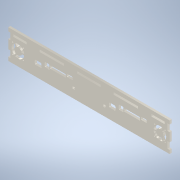
# Autodesk Inventor part: case bottom back
Saved by Autodesk Inventor 2022 (Build 260153000, 153)
## iProperties
Created: 2021-05-28
Part Number: case bottom back
Material: Titanium
Document SubType Name: Modeling
Designer: benka
Density: 4.51 g/cm^3
Appearance: Titanium
Author: benka
Autodesk Inventor part; units mm, degrees
ref_plane "YZ Plane" through (0, 0, 0) normal (1, 0, 0) x (0, 1, 0)
ref_plane "XZ Plane" through (0, 0, 0) normal (0, 1, 0) x (-1, 0, 0)
ref_plane "XY Plane" through (0, 0, 0) normal (0, 0, 1) x (1, 0, 0)
sketch "Sketch1" plane through (0, 0, 0) normal (0, 0, 1) x (1, 0, 0)
  circle A0 centre (-374.8345, 89.3147) radius 3
  line L0 (-376.9823, 107.1342) -> (-376.9823, 104.6342)
  line L1 (-378.9823, 102.6342) -> (-387.9823, 102.6342)
  line L2 (-389.9823, 104.6342) -> (-389.9823, 107.1342)
  line L3 (-392.0636, 104.796) -> (-392.0636, 101.796)
  line L4 (-394.0636, 99.796) -> (-426.0636, 99.796)
  line L5 (-428.0636, 101.796) -> (-428.0636, 104.796)
  line L6 (-429.4023, 105.6169) -> (-429.4023, 99.1169)
  line L7 (-431.4023, 97.1169) -> (-438.2023, 97.1169)
  line L8 (-440.2023, 99.1169) -> (-440.2023, 105.6169)
  line L9 (-447.5294, 98.9881) -> (-447.5294, 92.9881)
  line L10 (-460.5294, 100.9881) -> (-449.5294, 100.9881)
  line L11 (-449.5294, 90.9881) -> (-460.5294, 90.9881)
  line L12 (-462.5294, 92.9881) -> (-462.5294, 98.9881)
  circle A1 centre (-488.8435, 85.8263) radius 1.5
  circle A2 centre (-512.8435, 85.8263) radius 1.5
  circle A3 centre (-512.8435, 109.8263) radius 1.5
  circle A4 centre (-488.8435, 109.8263) radius 1.5
  arc A5 (-486.648, 100.2443) -> (-505.8473, 111.329) centre (-500.8435, 97.8263) ccw
  arc A6 (-505.8473, 111.329) -> (-506.3659, 109.8913) centre (-505.4999, 110.3913) ccw
  line L13 (-503.8384, 105.5136) -> (-506.3659, 109.8913)
  line L14 (-508.5309, 108.6413) -> (-506.0034, 104.2636)
  arc A7 (-508.5309, 108.6413) -> (-510.0353, 108.9111) centre (-509.397, 108.1413) ccw
  arc A8 (-510.0353, 108.9111) -> (-510.0353, 86.7416) centre (-500.8435, 97.8263) ccw
  arc A9 (-506.0034, 104.2636) -> (-506.0034, 91.3891) centre (-500.8435, 97.8263) ccw
  arc A10 (-492.6888, 99.0763) -> (-503.8384, 105.5136) centre (-500.8435, 97.8263) ccw
  line L15 (-487.6338, 99.0763) -> (-492.6888, 99.0763)
  arc A11 (-487.6338, 99.0763) -> (-486.648, 100.2443) centre (-487.6338, 100.0763) ccw
  line L16 (-492.6888, 96.5763) -> (-487.6338, 96.5763)
  arc A12 (-486.648, 95.4084) -> (-487.6338, 96.5763) centre (-487.6338, 95.5763) ccw
  arc A13 (-505.8473, 84.3237) -> (-486.648, 95.4084) centre (-500.8435, 97.8263) ccw
  arc A14 (-503.8384, 90.1391) -> (-492.6888, 96.5763) centre (-500.8435, 97.8263) ccw
  line L17 (-506.3659, 85.7614) -> (-503.8384, 90.1391)
  arc A15 (-506.3659, 85.7614) -> (-505.8473, 84.3237) centre (-505.4999, 85.2614) ccw
  line L18 (-506.0034, 91.3891) -> (-508.5309, 87.0114)
  arc A16 (-510.0353, 86.7416) -> (-508.5309, 87.0114) centre (-509.397, 87.5114) ccw
  line L19 (-438.2023, 107.6169) -> (-431.4023, 107.6169)
  line L20 (-426.0636, 106.796) -> (-394.0636, 106.796)
  line L21 (-387.9823, 109.1342) -> (-378.9823, 109.1342)
  arc A17 (-462.5294, 92.9881) -> (-460.5294, 90.9881) centre (-460.5294, 92.9881) ccw
  arc A18 (-449.5294, 90.9881) -> (-447.5294, 92.9881) centre (-449.5294, 92.9881) ccw
  arc A19 (-447.5294, 98.9881) -> (-449.5294, 100.9881) centre (-449.5294, 98.9881) ccw
  arc A20 (-460.5294, 100.9881) -> (-462.5294, 98.9881) centre (-460.5294, 98.9881) ccw
  arc A21 (-440.2023, 99.1169) -> (-438.2023, 97.1169) centre (-438.2023, 99.1169) ccw
  arc A22 (-431.4023, 97.1169) -> (-429.4023, 99.1169) centre (-431.4023, 99.1169) ccw
  arc A23 (-429.4023, 105.6169) -> (-431.4023, 107.6169) centre (-431.4023, 105.6169) ccw
  arc A24 (-438.2023, 107.6169) -> (-440.2023, 105.6169) centre (-438.2023, 105.6169) ccw
  arc A25 (-428.0636, 101.796) -> (-426.0636, 99.796) centre (-426.0636, 101.796) ccw
  arc A26 (-426.0636, 106.796) -> (-428.0636, 104.796) centre (-426.0636, 104.796) ccw
  arc A27 (-392.0636, 104.796) -> (-394.0636, 106.796) centre (-394.0636, 104.796) ccw
  arc A28 (-394.0636, 99.796) -> (-392.0636, 101.796) centre (-394.0636, 101.796) ccw
  arc A29 (-389.9823, 104.6342) -> (-387.9823, 102.6342) centre (-387.9823, 104.6342) ccw
  arc A30 (-387.9823, 109.1342) -> (-389.9823, 107.1342) centre (-387.9823, 107.1342) ccw
  arc A31 (-376.9823, 107.1342) -> (-378.9823, 109.1342) centre (-378.9823, 107.1342) ccw
  arc A32 (-378.9823, 102.6342) -> (-376.9823, 104.6342) centre (-378.9823, 104.6342) ccw
  line L22 (-522.8987, 75.8147) -> (-522.8987, 67.8147)
  line L23 (-522.8987, 75.8147) -> (-517.8987, 75.8147)
  line L24 (-517.8987, 90.8139) -> (-517.8987, 75.8147)
  line L25 (-522.8987, 90.8139) -> (-517.8987, 90.8139)
  line L26 (-522.8987, 110.8139) -> (-522.8987, 90.8139)
  line L27 (-522.8987, 110.8139) -> (-517.8987, 110.8139)
  line L28 (-522.8987, 125.8154) -> (-517.8987, 125.8154)
  line L29 (-522.8987, 125.8154) -> (-522.8987, 133.8154)
  line L30 (-161.8987, 125.8154) -> (-161.8987, 110.8139)
  line L31 (-161.8987, 110.8139) -> (-156.8987, 110.8139)
  line L32 (-156.8987, 110.8139) -> (-156.8987, 90.8139)
  line L33 (-161.8987, 90.8139) -> (-156.8987, 90.8139)
  line L34 (-161.8987, 90.8139) -> (-161.8987, 75.8147)
  line L35 (-161.8987, 75.8147) -> (-156.8987, 75.8147)
  line L36 (-156.8987, 75.8147) -> (-156.8987, 67.8147)
  line L37 (-161.8987, 125.8154) -> (-156.8987, 125.8154)
  line L38 (-156.8987, 125.8154) -> (-156.8987, 133.8154)
  line L39 (-156.8987, 133.8154) -> (-522.8987, 133.8154)
  line L40 (-522.8987, 67.8147) -> (-156.8987, 67.8147)
  line L41 (-511.3987, 125.8154) -> (-481.3987, 125.8154)
  line L42 (-481.3987, 120.8154) -> (-481.3987, 125.8154)
  line L43 (-511.3987, 120.8154) -> (-481.3987, 120.8154)
  line L44 (-511.3987, 120.8154) -> (-511.3987, 125.8154)
  line L45 (-451.3987, 125.8154) -> (-396.3987, 125.8154)
  line L46 (-451.3987, 120.8154) -> (-451.3987, 125.8154)
  line L47 (-451.3987, 120.8154) -> (-396.3987, 120.8154)
  line L48 (-396.3987, 120.8154) -> (-396.3987, 125.8154)
  line L49 (-366.3987, 120.8154) -> (-366.3987, 125.8154)
  line L50 (-366.3987, 125.8154) -> (-313.3987, 125.8154)
  line L51 (-366.3987, 120.8154) -> (-313.3987, 120.8154)
  line L52 (-313.3987, 120.8154) -> (-313.3987, 125.8154)
  line L53 (-283.3987, 120.8154) -> (-283.3987, 125.8154)
  line L54 (-283.3987, 125.8154) -> (-228.3987, 125.8154)
  line L55 (-283.3987, 120.8154) -> (-228.3987, 120.8154)
  line L56 (-228.3987, 120.8154) -> (-228.3987, 125.8154)
  line L57 (-198.3987, 120.8154) -> (-198.3987, 125.8154)
  line L58 (-198.3987, 125.8154) -> (-168.3987, 125.8154)
  line L59 (-168.3987, 120.8154) -> (-168.3987, 125.8154)
  line L60 (-198.3987, 120.8154) -> (-168.3987, 120.8154)
  circle A33 centre (-304.8345, 89.3147) radius 3
  line L61 (-187.1085, 96.5763) -> (-192.1635, 96.5763)
  line L62 (-192.1635, 99.0763) -> (-187.1085, 99.0763)
  arc A34 (-192.1635, 96.5763) -> (-193.1493, 95.4084) centre (-192.1635, 95.5763) ccw
  arc A35 (-193.1493, 100.2443) -> (-192.1635, 99.0763) centre (-192.1635, 100.0763) ccw
  circle A36 centre (-190.9538, 85.8263) radius 1.5
  circle A37 centre (-190.9538, 109.8263) radius 1.5
  arc A38 (-173.95, 111.329) -> (-193.1493, 100.2443) centre (-178.9538, 97.8263) ccw
  arc A39 (-193.1493, 95.4084) -> (-173.95, 84.3237) centre (-178.9538, 97.8263) ccw
  arc A40 (-175.9589, 105.5136) -> (-187.1085, 99.0763) centre (-178.9538, 97.8263) ccw
  arc A41 (-187.1085, 96.5763) -> (-175.9589, 90.1391) centre (-178.9538, 97.8263) ccw
  line L63 (-173.4314, 85.7614) -> (-175.9589, 90.1391)
  arc A42 (-173.95, 84.3237) -> (-173.4314, 85.7614) centre (-174.2975, 85.2614) ccw
  line L64 (-173.7939, 91.3891) -> (-171.2664, 87.0114)
  arc A43 (-171.2664, 87.0114) -> (-169.762, 86.7416) centre (-170.4003, 87.5114) ccw
  circle A44 centre (-166.9538, 85.8263) radius 1.5
  circle A45 centre (-166.9538, 109.8263) radius 1.5
  arc A46 (-173.4314, 109.8913) -> (-173.95, 111.329) centre (-174.2975, 110.3913) ccw
  line L65 (-175.9589, 105.5136) -> (-173.4314, 109.8913)
  line L66 (-171.2664, 108.6413) -> (-173.7939, 104.2636)
  arc A47 (-169.762, 108.9111) -> (-171.2664, 108.6413) centre (-170.4003, 108.1413) ccw
  arc A48 (-169.762, 86.7416) -> (-169.762, 108.9111) centre (-178.9538, 97.8263) ccw
  arc A49 (-173.7939, 91.3891) -> (-173.7939, 104.2636) centre (-178.9538, 97.8263) ccw
  line L67 (-259.9407, 101.6096) -> (-259.9407, 104.6096)
  line L68 (-225.9407, 99.6096) -> (-257.9407, 99.6096)
  line L69 (-257.9407, 106.6096) -> (-225.9407, 106.6096)
  line L70 (-223.9407, 104.6096) -> (-223.9407, 101.6096)
  line L71 (-221.7993, 104.5587) -> (-221.7993, 107.0587)
  line L72 (-210.7993, 102.5587) -> (-219.7993, 102.5587)
  line L73 (-208.7993, 107.0587) -> (-208.7993, 104.5587)
  arc A50 (-281.5589, 91.018) -> (-279.5589, 93.018) centre (-281.5589, 93.018) ccw
  line L74 (-279.5589, 99.018) -> (-279.5589, 93.018)
  line L75 (-292.5589, 101.018) -> (-281.5589, 101.018)
  line L76 (-294.5589, 93.018) -> (-294.5589, 99.018)
  line L77 (-281.5589, 91.018) -> (-292.5589, 91.018)
  line L78 (-219.7993, 109.0587) -> (-210.7993, 109.0587)
  arc A51 (-279.5589, 99.018) -> (-281.5589, 101.018) centre (-281.5589, 99.018) ccw
  arc A52 (-294.5589, 93.018) -> (-292.5589, 91.018) centre (-292.5589, 93.018) ccw
  arc A53 (-257.9407, 106.6096) -> (-259.9407, 104.6096) centre (-257.9407, 104.6096) ccw
  arc A54 (-259.9407, 101.6096) -> (-257.9407, 99.6096) centre (-257.9407, 101.6096) ccw
  arc A55 (-292.5589, 101.018) -> (-294.5589, 99.018) centre (-292.5589, 99.018) ccw
  arc A56 (-225.9407, 99.6096) -> (-223.9407, 101.6096) centre (-225.9407, 101.6096) ccw
  arc A57 (-223.9407, 104.6096) -> (-225.9407, 106.6096) centre (-225.9407, 104.6096) ccw
  arc A58 (-221.7993, 104.5587) -> (-219.7993, 102.5587) centre (-219.7993, 104.5587) ccw
  arc A59 (-219.7993, 109.0587) -> (-221.7993, 107.0587) centre (-219.7993, 107.0587) ccw
  arc A60 (-210.7993, 102.5587) -> (-208.7993, 104.5587) centre (-210.7993, 104.5587) ccw
  arc A61 (-208.7993, 107.0587) -> (-210.7993, 109.0587) centre (-210.7993, 107.0587) ccw
  line L79 (-517.8987, 110.8139) -> (-517.8987, 125.8154)
  line L80 (-261.4498, 105.7999) -> (-261.4498, 99.2999)
  line L81 (-263.4498, 97.2999) -> (-270.2498, 97.2999)
  line L82 (-272.2498, 99.2999) -> (-272.2498, 105.7999)
  line L83 (-270.2498, 107.7999) -> (-263.4498, 107.7999)
  arc A62 (-270.2498, 107.7999) -> (-272.2498, 105.7999) centre (-270.2498, 105.7999) ccw
  arc A63 (-272.2498, 99.2999) -> (-270.2498, 97.2999) centre (-270.2498, 99.2999) ccw
  arc A64 (-261.4498, 105.7999) -> (-263.4498, 107.7999) centre (-263.4498, 105.7999) ccw
  arc A65 (-263.4498, 97.2999) -> (-261.4498, 99.2999) centre (-263.4498, 99.2999) ccw
  point P0 (-447.5294, 100.9881)
  point P1 (-447.5294, 90.9881)
  point P2 (-462.5294, 100.9881)
  point P3 (-462.5294, 90.9881)
  point P4 (-279.5589, 91.018)
  point P5 (-279.5589, 101.018)
  point P6 (-294.5589, 101.018)
  point P7 (-294.5589, 91.018)
  dimension "d74" = 15
  dimension "d75" = 10
  dimension "d78" = 7
  dimension "d79" = 36
  dimension "d80" = 13
  dimension "d81" = 6.5
  dimension "d82" = 2
  dimension "d83" = 2
  dimension "d87" = 70
  dimension "d88" = 366
  dimension "d89" = 10.5
  dimension "d90" = 10.8
  dimension "d91" = 15
  dimension "d92" = 10
  dimension "d93" = 10.5
  dimension "d94" = 10.8
  dimension "d95" = 21.5
  dimension "d96" = 21.5
  constraints: 168 end point, 112 point on circle, 66 centre point, 64 tangent, 27 equal radius, 20 vertical, 18 horizontal, 16 point on line, 14 parallel, 9 perpendicular, 2 coincident, 38 other
  measures "d74" distance between parallel lines of L74 L76
  measures "d75" distance between parallel lines of L77 L75
  measures "d78" distance between parallel lines of L69 L68
  measures "d79" distance between parallel lines of L70 L67
  measures "d80" distance between parallel lines of L73 L71
  measures "d81" distance between parallel lines of L72 L78
  measures "d82" radius of A52
  measures "d83" radius of A54
  measures "d87" distance of point (-304.834, 89.315) point (-374.834, 89.315)
  measures "d88" distance between parallel lines of L36 L22
  measures "d89" distance between parallel lines of L83 L81
  measures "d90" distance between parallel lines of L82 L80
  measures "d91" distance between parallel lines of L12 L9
  measures "d92" distance between parallel lines of L10 L11
  measures "d93" distance between parallel lines of L19 L7
  measures "d94" distance between parallel lines of L6 L8
  measures "d95" distance from line of L40 A0.centre
  measures "d96" distance from line of L40 A33.centre
extrude "Extrusion1" add sketch "Sketch1" along normal blind 5
body "Solid1"
